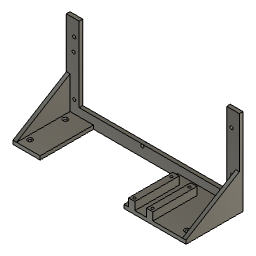
Display_Mount (Autodesk Fusion 360 design; units mm, degrees)
Autodesk Fusion 360 part; units mm, degrees
sketch "Master" plane through (0, 0, 0) normal (0, 1, 0) x (1, 0, 0)
  line L0 (0, 0) -> (-191.2, 0)
  line L1 (-191.2, 0) -> (-191.2, 95.5)
  line L2 (-191.2, 95.5) -> (0, 95.5) construction
  line L3 (0, 95.5) -> (0, 0)
  circle A0 centre (-8.75, 17.825) radius 1.65 construction
  line L4 (-14.1, 12.75) -> (-177.1, 12.75)
  line L5 (-177.1, 12.75) -> (-177.1, 82.75)
  line L6 (-177.1, 82.75) -> (-14.1, 82.75) construction
  line L7 (-14.1, 82.75) -> (-14.1, 12.75)
  line L8 (-95.6, 12.75) -> (-95.6, 0) construction
  line L9 (-14.1, 47.75) -> (0, 47.75) construction
  line L10 (-8.75, 17.825) -> (-8.75, 77.675) construction
  circle A1 centre (-8.75, 77.675) radius 1.65 construction
  circle A2 centre (-182.45, 17.825) radius 1.65 construction
  circle A3 centre (-182.45, 77.675) radius 1.65 construction
  circle A4 centre (-183.2, 63) radius 1.2 construction
  circle A5 centre (-8, 32.5) radius 1.2 construction
  circle A6 centre (-107.2, 10.85) radius 1.65 construction
  circle A7 centre (-84, 84.65) radius 1.65 construction
  line L11 (-68.6, 16.75) -> (-24.1, 16.75) construction
  line L12 (-24.1, 16.75) -> (-24.1, 18.35) construction
  line L13 (-24.1, 18.35) -> (-68.6, 18.35) construction
  line L14 (-68.6, 18.35) -> (-68.6, 16.75) construction
  line L15 (-68.6, 16.75) -> (-24.1, 16.75) construction
  line L16 (-24.1, 16.75) -> (-24.1, 7.75) construction
  line L17 (-24.1, 7.75) -> (-68.6, 7.75) construction
  line L18 (-68.6, 7.75) -> (-68.6, 16.75) construction
  line L19 (-68.6, 18.35) -> (-24.1, 18.35) construction
  line L20 (-24.1, 18.35) -> (-24.1, 38.35) construction
  line L21 (-24.1, 38.35) -> (-68.6, 38.35) construction
  line L22 (-68.6, 38.35) -> (-68.6, 18.35) construction
  line L23 (-191.2, 95.5) -> (-177.1, 95.5)
  line L24 (-177.1, 95.5) -> (-177.1, 82.75)
  line L25 (-14.1, 82.75) -> (-14.1, 95.5)
  line L26 (-14.1, 95.5) -> (0, 95.5)
  circle A8 centre (-8.75, 77.675) radius 1.75
  circle A9 centre (-8.75, 17.825) radius 1.75
  circle A10 centre (-107.2, 10.85) radius 1.75
  circle A11 centre (-182.45, 17.825) radius 1.75
  circle A12 centre (-182.45, 77.675) radius 1.75
  circle A13 centre (-8, 32.5) radius 1.75
  circle A14 centre (-183.2, 63) radius 1.75
  line L27 (-68.6, 12.75) -> (-68.6, 0)
  line L28 (-14.1, 40) -> (0, 40)
  line L29 (-68.6, 4) -> (-4, 4)
  line L30 (-4, 4) -> (-4, 40)
  line L31 (-63.45, 4) -> (-63.45, 16.75)
  line L32 (-63.45, 16.75) -> (-56.45, 16.75)
  line L33 (-56.45, 16.75) -> (-56.45, 4)
  line L34 (-43.65, 4) -> (-43.65, 16.75)
  line L35 (-43.65, 16.75) -> (-36.65, 16.75)
  line L36 (-36.65, 16.75) -> (-36.65, 4)
  line L37 (-68.6, 0) -> (-68.6, 4)
  line L38 (-68.6, 4) -> (-187.2, 4)
  line L39 (-187.2, 4) -> (-187.2, 40)
  line L40 (-187.2, 40) -> (-191.2, 40)
  line L41 (-161.2, 4) -> (-161.2, 0)
  point P0 (-40.15, 16.75)
  dimension "d1" = 191.2
  dimension "d2" = 95.5
  dimension "d3" = 163
  dimension "d4" = 70
  dimension "d5" = 59.85
  dimension "d6" = 8.75
  dimension "d7" = 3.3
  dimension "d8" = 8
  dimension "d9" = 32.5
  dimension "d10" = 2.4
  dimension "d11" = 8
  dimension "d12" = 32.5
  dimension "d13" = 10.85
  dimension "d14" = 10.85
  dimension "d15" = 84
  dimension "d16" = 84
  dimension "d21" = 44.5
  dimension "d22" = 1.6
  dimension "d23" = 9
  dimension "d24" = 20
  dimension "d26" = 4
  dimension "d28" = 3.5
  dimension "d29" = 3.5
  dimension "d32" = 10
  dimension "d33" = 7.5
  dimension "d36" = 4
  dimension "d37" = 4
  dimension "d38" = 7
  dimension "d39" = 7
  dimension "d40" = 16.05
  dimension "d41" = 19.8
  dimension "d47" = 4
  dimension "d63" = 30
  constraint horizontal L0
  constraint vertical L1
  constraint horizontal L2
  constraint vertical L3
  constraint coincident L0.start L3.end
  constraint horizontal L4
  constraint vertical L5
  constraint horizontal L6
  constraint vertical L7
  constraint midpoint L4 L8.start
  constraint midpoint L0 L8.end
  constraint midpoint L7 L9.start
  constraint midpoint L3 L9.end
  constraint horizontal L9
  constraint vertical L8
  constraint coincident A0.centre L10.start
  constraint parallel L3 L10
  constraint coincident L10.end A1.centre
  constraint equal A0 A1
  constraint symmetric A0.centre L9 L10.end
  constraint symmetric A0.centre L8 A2.centre
  constraint symmetric L8 L10.end A3.centre
  constraint equal A2 A3
  constraint equal A0 A3
  constraint equal A4 A5
  constraint equal A2 A6
  constraint equal A6 A7
  constraint horizontal L11
  constraint vertical L12
  constraint horizontal L13
  constraint vertical L14
  constraint horizontal L15
  constraint vertical L16
  constraint horizontal L17
  constraint vertical L18
  constraint coincident L11.end L12.start
  constraint horizontal L19
  constraint vertical L20
  constraint horizontal L21
  constraint vertical L22
  constraint coincident L12.end L13.start
  constraint coincident L2 L23.end
  constraint vertical L24
  constraint coincident L2 L25.end
  constraint perpendicular L2 L25
  constraint concentric A1 A8
  constraint concentric A0 A9
  constraint concentric A6 A10
  constraint concentric A2 A11
  constraint concentric A3 A12
  constraint equal A11 A12
  constraint equal A10 A11
  constraint equal A9 A10
  constraint equal A8 A9
  constraint concentric A5 A13
  constraint concentric A4 A14
  constraint equal A13 A14
  constraint coincident L4 L27.start
  constraint coincident L18 L27.start
  constraint coincident L0 L27.end
  constraint perpendicular L0 L27
  constraint coincident L7 L28.start
  constraint coincident L3 L28.end
  constraint perpendicular L3 L28
  constraint coincident L27 L29.start
  constraint perpendicular L27 L29
  constraint coincident L28 L30.end
  constraint perpendicular L28 L30
  constraint coincident L29 L31.start
  constraint coincident L15 L31.end
  constraint perpendicular L15 L31
  constraint coincident L15 L32.end
  constraint coincident L29 L33.end
  constraint perpendicular L29 L33
  constraint coincident L29 L34.start
  constraint coincident L11 L34.end
  constraint perpendicular L11 L34
  constraint coincident L11 L35.end
  constraint coincident L29 L36.end
  constraint perpendicular L29 L36
  constraint midpoint L35 P0
  constraint perpendicular L0 L37
  constraint perpendicular L37 L38
  constraint perpendicular L0 L39
  constraint coincident L1 L40.end
  constraint perpendicular L1 L40
  constraint collinear L28 L40
  constraint collinear L29 L38
  constraint coincident L29.start L37.end
  constraint coincident L38 L41.start
  constraint coincident L0 L41.end
  constraint perpendicular L0 L41
  measures "d1" distance of L0.start L0.end
  measures "d2" distance of L0.start L2.end
  measures "d3" distance of L4.start L4.end
  measures "d4" distance of L4.start L6.end
  measures "d5" distance of A0.centre L10.end
  measures "d6" horizontal distance of L2.end L10.end
  measures "d7" diameter of A1
  measures "d8" distance of L1 A4.centre
  measures "d9" vertical distance of L1.end A4.centre
  measures "d10" diameter of A4
  measures "d11" distance of L3 A5.centre
  measures "d12" distance of L0 A5.centre
  measures "d13" distance of L0 A6.centre
  measures "d14" distance of L2 A7.centre
  measures "d15" distance of L1 A6.centre
  measures "d16" horizontal distance of L2.end A7.centre
  measures "d21" distance of L12.end L13.end
  measures "d22" distance of L11.end L12.end
  measures "d23" distance of L11.end L16.end
  measures "d24" distance of L12.end L20.end
  measures "d26" vertical distance of L4.end L11.start
  measures "d28" diameter of A12
  measures "d29" diameter of A14
  measures "d32" horizontal distance of L4.start L11.end
  measures "d33" vertical distance of A5.centre L28.end
  measures "d36" distance of L0 L29
  measures "d37" distance of L3 L30
  measures "d38" distance of L34.start L36.end
  measures "d39" distance of L31.start L33.end
  measures "d40" distance of L11.end P0
  measures "d41" distance of L32.end L35.end
  measures "d47" horizontal distance of L0.end L38.end
  measures "d63" distance of L0.end L41.end
sketch "Schablone" plane through (0, 0, 0) normal (0, 1, 0) x (1, 0, 0)
  line L0 (-191.2, 0) -> (0, 0)
  line L1 (0, 0) -> (0, 95.5)
  line L2 (0, 95.5) -> (-191.2, 95.5)
  line L3 (-191.2, 95.5) -> (-191.2, 0)
  line L4 (-177.1, 12.75) -> (-14.1, 12.75)
  line L5 (-14.1, 12.75) -> (-14.1, 82.75)
  line L6 (-14.1, 82.75) -> (-177.1, 82.75)
  line L7 (-177.1, 82.75) -> (-177.1, 12.75)
  circle A0 centre (-182.45, 17.825) radius 2.65
  circle A1 centre (-107.2, 10.85) radius 2.65
  circle A2 centre (-182.45, 77.675) radius 2.65
  circle A3 centre (-183.2, 63) radius 1.75
  circle A4 centre (-83.8424, 84.5376) radius 2.65
  circle A5 centre (-8.75, 17.825) radius 2.65
  circle A6 centre (-8, 32.5) radius 1.75
  circle A7 centre (-8.75, 77.675) radius 2.65
  point P0 (-14.1, 12.75)
  point P1 (-191.2, 95.5)
  point P2 (-177.1, 82.75)
  point P3 (-182.45, 77.675)
  point P4 (-183.2, 63)
  point P5 (-182.45, 17.825)
  point P6 (-107.2, 10.85)
  point P7 (-8.75, 17.825)
  point P8 (-8, 32.5)
  point P9 (-8.75, 77.675)
  dimension "d17" = 5.3
  dimension "d18" = 3.5
  constraint horizontal L0
  constraint vertical L1
  constraint horizontal L2
  constraint vertical L3
  constraint horizontal L4
  constraint vertical L5
  constraint horizontal L6
  constraint vertical L7
  constraint coincident L0.end L1.start
  constraint coincident P0 L4.end
  constraint coincident P1 L2.end
  constraint coincident P2 L6.end
  constraint coincident P3 A2.centre
  constraint coincident P4 A3.centre
  constraint coincident P5 A0.centre
  constraint coincident P6 A1.centre
  constraint coincident P7 A5.centre
  constraint coincident P8 A6.centre
  constraint coincident P9 A7.centre
  constraint equal A1 A5
  constraint equal A0 A1
  constraint equal A0 A2
  constraint equal A2 A4
  constraint equal A4 A7
  constraint equal A3 A6
  measures "d17" diameter of A7
  measures "d18" diameter of A6
extrude "Extrude1" add sketch "Schablone" along normal blind 0.4 makes body 1
extrude "Extrude2" add sketch "Master" along normal blind 4 separate body contours L0 L3 L27 L28 L29 L30 L37 | L0 L27 L37 L38 L41 | L3 L7 L25 L26 L28 | L0 L1 L38 L39 L40 L41 | L1 L4 L5 L23 L24 L27 L38 L39 L40 | L4 L27 L29 L31 | L4 L7 L28 L29 L30 L36 | L4 L29 L31 L33 | L4 L29 L33 L34 | L4 L29 L34 L36 makes body 2
extrude "Extrude3" add sketch "Master" along normal blind 63 contours L0 L3 L27 L28 L29 L30 L37 | L0 L1 L38 L39 L40 L41 | L4 L29 L31 L33 | L4 L29 L34 L36 bodies 2
sketch "Sketch3" plane through (0, 0, -12.75) normal (0, 0, -1) x (1, 0, 0)
  line L0 (-14.1, 0) -> (-177.1, 0)
  line L1 (-177.1, 0) -> (-177.1, -4)
  line L2 (-177.1, -4) -> (-63.45, -4)
  line L3 (-63.45, -4) -> (-63.45, -63)
  line L4 (-63.45, -63) -> (-56.45, -63)
  line L5 (-56.45, -63) -> (-56.45, -4)
  line L6 (-56.45, -4) -> (-43.65, -4)
  line L7 (-43.65, -4) -> (-43.65, -63)
  line L8 (-43.65, -63) -> (-36.65, -63)
  line L9 (-36.65, -63) -> (-36.65, -4)
  line L10 (-36.65, -4) -> (-14.1, -4)
  line L11 (-14.1, -4) -> (-14.1, 0)
  circle A0 centre (-59.95, -59.8) radius 1.4
  circle A1 centre (-40.15, -59.8) radius 1.4
  line L12 (-63.45, -4) -> (-56.45, -4)
  line L13 (-59.95, -4) -> (-59.95, -59.8) construction
  line L14 (-40.15, -4) -> (-40.15, -59.8) construction
  circle A2 centre (-59.95, -19.15) radius 1.4
  circle A3 centre (-40.15, -19.15) radius 1.4
  line L15 (-59.95, -19.15) -> (-40.15, -19.15) construction
  line L16 (-59.95, -59.8) -> (-40.15, -59.8) construction
  line L17 (-43.65, -4) -> (-36.65, -4)
  line L18 (-63.45, -14.15) -> (-56.45, -14.15)
  line L19 (-43.65, -14.15) -> (-36.65, -14.15)
  dimension "d42" = 15.15
  dimension "d43" = 40.65
  dimension "d44" = 2.8
  dimension "d60" = 5
  constraint coincident L2.end L3.start
  constraint coincident L5.end L6.start
  constraint midpoint L12 L13.start
  constraint coincident A0.centre L13.end
  constraint coincident A1.centre L14.end
  constraint vertical L13
  constraint vertical L14
  constraint coincident L13 A2.centre
  constraint coincident L14 A3.centre
  constraint coincident A2.centre L15.start
  constraint coincident A3.centre L15.end
  constraint horizontal L15
  constraint horizontal L16
  constraint equal A2 A3
  constraint equal A1 A3
  constraint equal A0 A1
  constraint coincident L6.end L7.start
  constraint coincident L9.end L10.start
  constraint midpoint L14.start L17
  constraint coincident L3 L18.start
  constraint coincident L5 L18.end
  constraint perpendicular L5 L18
  constraint coincident L7 L19.start
  constraint coincident L9 L19.end
  constraint perpendicular L9 L19
  constraint collinear L18 L19
  measures "d42" distance of L14.start A3.centre
  measures "d43" distance of A1.centre A3.centre
  measures "d44" diameter of A2
  measures "d60" vertical distance of A2.centre L18.start
extrude "Extrude8" cut sketch "Sketch3" against normal up to surface (8.75 mm away) contours L7 L9 L17 L19 | L3 L5 L12 L18 bodies 2
extrude "Extrude4" cut sketch "Sketch3" against normal blind 9 contours A0 | A1 | A2 | A3 bodies 2
sketch "Sketch4" plane through (0, 0, -4) normal (0, 0, -1) x (1, 0, 0)
  line L0 (-4, -4) -> (-68.6, -4)
  line L1 (-36.65, -14.15) -> (-36.65, -63)
  line L2 (-68.6, -63) -> (-63.45, -63)
  line L3 (-4, -63) -> (-4, -4)
  circle A0 centre (-9, -14) radius 1.75
  circle A1 centre (-9, -53) radius 1.75
  circle A2 centre (-182.2, -53) radius 1.75
  circle A3 centre (-182.2, -14) radius 1.75
  line L4 (-9, -53) -> (-182.2, -53) construction
  line L5 (-182.2, -53) -> (-182.2, -14) construction
  line L6 (-182.2, -14) -> (-9, -14) construction
  line L7 (-9, -14) -> (-9, -53) construction
  line L8 (-187.2, -4) -> (-187.2, -63) construction
  line L9 (-63.45, -63) -> (-63.45, -14.15)
  line L10 (-63.45, -14.15) -> (-56.45, -14.15)
  line L11 (-56.45, -14.15) -> (-56.45, -63)
  line L12 (-56.45, -63) -> (-43.65, -63)
  line L13 (-43.65, -63) -> (-43.65, -14.15)
  line L14 (-43.65, -14.15) -> (-36.65, -14.15)
  line L15 (-36.65, -63) -> (-4, -63)
  line L16 (-68.6, -4) -> (-68.6, -63)
  dimension "d48" = 5
  dimension "d49" = 5
  dimension "d50" = 10
  dimension "d51" = 10
  dimension "d52" = 3.5
  constraint horizontal L4
  constraint vertical L5
  constraint horizontal L6
  constraint vertical L7
  constraint coincident A3.centre L5.end
  constraint coincident A1.centre L4.start
  constraint coincident A2.centre L4.end
  constraint coincident A0.centre L6.end
  constraint equal A1 A2
  constraint equal A0 A2
  constraint equal A0 A3
  measures "d48" distance of L3 L7
  measures "d49" distance of A2.centre L8
  measures "d50" distance of L6 L8.start
  measures "d51" vertical distance of A2.centre L8.end
  measures "d52" diameter of A2
extrude "Extrude5" cut sketch "Sketch4" against normal blind 13 contours A0 | A1 | A2 | A3 bodies 2
chamfer "Chamfer1" distance 1 angle 45 4 edges at (-10.6316, 52.3672, -4) (-10.6316, 13.3672, -4) (-183.8316, 52.3672, -4) (-183.8316, 13.3672, -4) on bodies 2
sketch "Sketch5" plane through (-4, 0, 0) normal (-1, 0, 0) x (0, -1, 0)
  line L0 (-4, -40) -> (-4, -4)
  line L1 (-4, -4) -> (-63, -4)
  line L2 (-63, -4) -> (-63, -40)
  line L3 (-63, -40) -> (-4, -40)
  line L4 (-63, -4) -> (-4, -40)
  constraint coincident L1.end L2.start
  constraint coincident L0.start L3.end
extrude "Extrude6" cut sketch "Sketch5" against normal blind 65 contours L2 L3 L4 bodies 2
sketch "Sketch6" plane through (-187.2, 0, 0) normal (1, 0, 0) x (0, 1, 0)
  line L0 (4, -4) -> (4, -40)
  line L1 (4, -40) -> (63, -40)
  line L2 (63, -40) -> (63, -4)
  line L3 (4, -40) -> (63, -4)
  line L4 (63, -4) -> (4, -4)
  constraint coincident L0.end L1.start
  constraint coincident L2.end L3.end
extrude "Extrude7" cut sketch "Sketch6" against normal blind 59 contours L1 L2 L3 bodies 2
move_body "Move1" bodies 2 to x (1, 0, 0) y (0, -1, 0) z (0, 0, -1) at (0, 0, -191)
hidden bodies 1
equation "d5 = ( ( 64.7 + 55 ) / 2 ) * 1 mm"
equation "d6 = ( ( 7.2 + 10.3 ) / 2 ) * 1 mm"
equation "d11 = d8"
equation "d12 = d9"
equation "d13 = ( ( 9.2 + 12.5 ) / 2 ) * 1 mm"
equation "d14 = d13"
equation "d16 = d15"
equation "d39 = d38"
equation "d40 = ( ( 14.7 + 17.4 ) / 2 ) * 1 mm"
equation "d42 = ( ( 13.8 + 16.5 ) / 2 ) * 1 mm"
equation "d43 = ( ( 43.2 + 38.1 ) / 2 ) * 1 mm"
equation "d47 = d37"
named bodies: "schablone"
